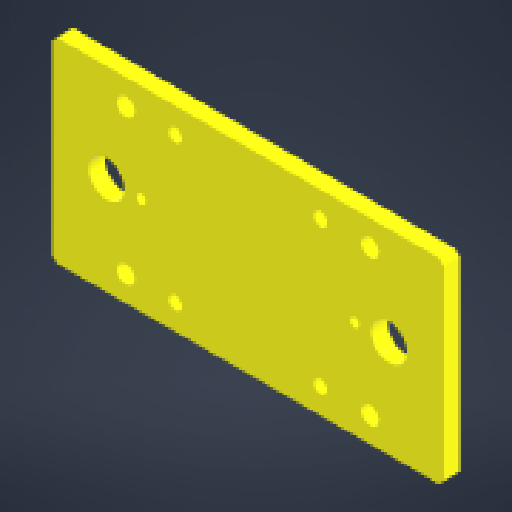
# Autodesk Inventor part: TilesGrip
Saved by Autodesk Inventor 2025 (Build 290162000, 162)
## iProperties
Created: 2024-05-26
Part Number: TilesGrip
Material: Generic
Document SubType Name: Modeling
Designer: zulet
Density: 1 g/cm^3
Appearance: Smooth - Yellow
Author: zulet
Autodesk Inventor part; units mm, degrees
ref_plane "YZ Plane" through (0, 0, 0) normal (1, 0, 0) x (0, 1, 0)
ref_plane "XZ Plane" through (0, 0, 0) normal (0, 1, 0) x (-1, 0, 0)
ref_plane "XY Plane" through (0, 0, 0) normal (0, 0, 1) x (1, 0, 0)
sketch "Sketch1" plane through (0, 0, 0) normal (0, 0, 1) x (1, 0, 0)
  circle A0 centre (-86.5, 0) radius 11 projected
  circle A1 centre (86.5, 0) radius 11 projected
  circle A2 centre (-75, 44.5) radius 5.5 projected
  circle A3 centre (-75, -44.5) radius 5.5 projected
  circle A4 centre (75, 44.5) radius 5.5 projected
  circle A5 centre (75, -44.5) radius 5.5 projected
  circle A6 centre (-65.5, 0) radius 3 projected
  circle A7 centre (65.5, 0) radius 3 projected
  circle A8 centre (-44.5, 44.5) radius 4.1881 projected
  circle A9 centre (-44.5, -44.5) radius 4.1881 projected
  circle A10 centre (44.5, 44.5) radius 4.1881 projected
  circle A11 centre (44.5, -44.5) radius 4.1881 projected
  line L0 (100, -58) -> (98, -60) construction
  line L1 (100, 58) -> (100, -58) construction
  line L2 (98, 60) -> (100, 58) construction
  line L3 (-98, 60) -> (98, 60) projected
  line L4 (-100, 58) -> (-98, 60) construction
  line L5 (-100, -58) -> (-100, 58) construction
  line L6 (-98, -60) -> (-100, -58) construction
  line L7 (98, -60) -> (-98, -60) projected
  line L8 (98, 60) -> (119, 60)
  line L9 (122, 57) -> (122, -57)
  line L10 (119, -60) -> (98, -60)
  line L11 (98, -60) -> (98, 60) construction
  line L12 (-98, 60) -> (-119, 60)
  line L13 (-122, 57) -> (-122, -57)
  line L14 (-119, -60) -> (-98, -60)
  line L15 (-98, -60) -> (-98, 60) construction
  line L16 (119, 60) -> (122, 57)
  line L17 (119, -60) -> (122, -57)
  line L18 (-122, -57) -> (-119, -60)
  line L19 (-122, 57) -> (-119, 60)
  point P0 (0, 0)
  point P1 (122, -60)
  point P2 (122, 60)
  point P3 (-122, -60)
  point P4 (-122, 60)
  dimension "d4" = 3
  dimension "d5" = 3
  dimension "d6" = 3
  dimension "d7" = 3
  dimension "d8" = 3
  dimension "d9" = 3
  dimension "d10" = 3
  dimension "d11" = 3
  dimension "d12" = 22
  dimension "d13" = 22
  constraints: 24 end point, 10 point on line, 4 parallel, 2 horizontal, 2 perpendicular
  measures "d4" distance of L8.end point (122, 60)
  measures "d5" distance of L9.start point (122, 60)
  measures "d6" distance of L10.start point (122, -60)
  measures "d7" distance of L9.end point (122, -60)
  measures "d8" distance of L13.end point (-122, -60)
  measures "d9" distance of L14.start point (-122, -60)
  measures "d10" distance of L13.start point (-122, 60)
  measures "d11" distance of L12.end point (-122, 60)
  measures "d12" distance between parallel lines of L13 L5
  measures "d13" distance between parallel lines of L1 L9
extrude "Extrusion1" add sketch "Sketch1" along normal blind 10
equation "\"d5\" = d4"
equation "\"d6\" = d4"
equation "\"d7\" = d6"
equation "\"d8\" = d4"
equation "\"d9\" = d8"
equation "\"d10\" = d4"
equation "\"d11\" = d10"
equation "\"d13\" = d12"
body "Solid1"
